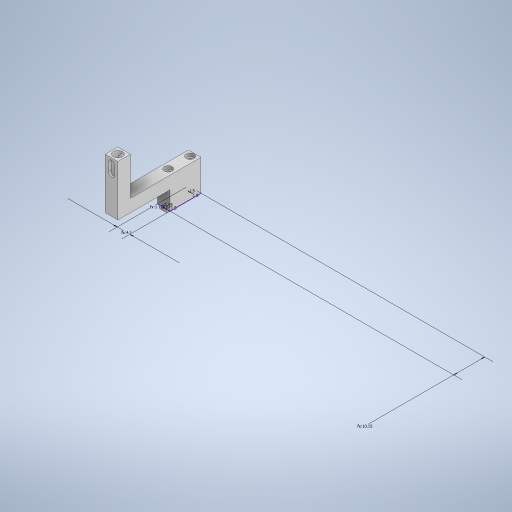
# Autodesk Inventor part: original_holder
Saved by Autodesk Inventor 2024 (Build 280153000, 153)
## iProperties
Created: 2023-05-03
Part Number: original_holder
Material: Generic
Document SubType Name: Modeling
Designer: Rober
Mass: 538.313 g
Surface Area: 676.575 cm^2
Volume: 538.313 cm^3
Density: 1 g/cm^3
Appearance: Default
Author: Rober
Autodesk Inventor part; units mm, degrees
ref_plane "YZ Plane" through (0, 0, 0) normal (1, 0, 0) x (0, 1, 0)
ref_plane "XZ Plane" through (0, 0, 0) normal (0, 1, 0) x (-1, 0, 0)
ref_plane "XY Plane" through (0, 0, 0) normal (0, 0, 1) x (1, 0, 0)
sketch "Sketch1" plane through (0, 0, 0) normal (0, 1, 0) x (-1, 0, 0)
  line L0 (-2.05, -5.575) -> (-6.15, -5.575)
  line L1 (-6.15, -5.575) -> (-6.15, 4.575)
  line L2 (-6.15, 4.575) -> (-2.05, 4.575)
  line L3 (-2.05, 4.575) -> (-2.05, -5.575)
  line L4 (-3.175, 4.575) -> (-5.025, 4.575)
  line L5 (-3.175, 4.575) -> (-3.175, -5.575)
  line L6 (-5.025, 4.575) -> (-5.025, -5.575)
  circle A0 centre (-4.1, 3.075) radius 0.75
  circle A1 centre (-4.1, -4.075) radius 0.75
  point P0 (-4.1, 4.575)
  point P1 (-4.1, -5.575)
  point P2 (-1.1679, -0.0702)
  point P3 (-4.1, 4.575)
  dimension "d13" = 4.1
  dimension "d14" = 10.15
  dimension "d44" = 1.85
  dimension "d45" = 1.125
  dimension "d46" = 1.5
  dimension "d47" = 1.5
  dimension "d48" = 1.5
  dimension "d49" = 1.5
  constraints: 14 end point, 4 point on line, 3 midpoint, 3 perpendicular, 2 centre point, 2 parallel, 1 horizontal
  measures "d13" distance of L0.start L0.end
  measures "d14" distance of point (-4.1, 4.575) point (-4.1, -5.575)
  measures "d44" distance of L4.start L4.end
  measures "d45" distance from line of L3 L4.start
  measures "d46" diameter of A0
  measures "d47" diameter of A1
  measures "d48" distance of point (-4.1, 4.575) A0.centre
  measures "d49" distance of point (-4.1, -5.575) A1.centre
extrude "Extrusion1" add sketch "Sketch1" along normal blind 10.15
sketch "Sketch11" plane through (2.05, 0, 4.575) normal (0, 0, 1) x (1, 0, 0)
  point P0 (-2.05, 0)
extrude "Extrusion6" add sketch "Sketch1" against normal blind 1 contours L0 L6 L2 L5
sketch "Sketch12" plane through (0, 10.15, 0) normal (0, 1, 0) x (1, 0, 0)
  circle A0 centre (4.0754, 4.0842) radius 1.265
  circle A1 centre (4.0754, -3.0807) radius 1.265
  point P0 (0, 0)
  dimension "d52" = 2.53
  dimension "d53" = 2.53
  constraints: 2 centre point
  measures "d52" diameter of A0
  measures "d53" diameter of A1
extrude "Extrusion7" cut sketch "Sketch12" against normal blind 1
sketch "Sketch13" plane through (2.05, 10.15, 4.575) normal (0, 0, 1) x (1, 0, 0)
  line L0 (0, 0) -> (0, -4.15)
  line L1 (0, -10.15) -> (0, 0) projected
  line L2 (0, -4.15) -> (4.1, -4.15)
  line L3 (4.1, -10.15) -> (4.1, 0) projected
  line L4 (4.1, 0) -> (4.1, -4.15)
  line L5 (0, 0) -> (4.1, 0)
  point P0 (-2.05, -10.15)
  dimension "d56" = 4.15
  constraints: 8 end point, 3 perpendicular, 2 point on line
  measures "d56" distance of L0.start L0.end
extrude "Extrusion8" add sketch "Sketch13" along normal blind 17
sketch "Sketch14" plane through (0, 10.15, 0) normal (0, 1, 0) x (1, 0, 0)
  line L0 (6.15, 5.575) -> (6.15, -21.575) projected
  line L1 (6.15, -21.575) -> (6.15, -17.465)
  line L2 (6.15, -17.465) -> (2.05, -17.465)
  line L3 (2.05, 5.575) -> (2.05, -21.575) projected
  line L4 (2.05, -21.575) -> (6.15, -21.575)
  point P0 (0, 0)
  dimension "d59" = 4.11
  constraints: 6 end point, 2 point on line, 1 parallel, 1 perpendicular
  measures "d59" distance of L0.end L1.end
extrude "Extrusion9" add sketch "Sketch14" along normal blind 12.4
sketch "Sketch15" plane through (2.05, 10.15, 21.575) normal (0, 0, 1) x (1, 0, 0)
  line L0 (2.05, 10.7632) -> (2.05, 7.9632) construction
  line L1 (4.1, 0) -> (4.1, 12.4) projected
  line L2 (1.05, 10.7632) -> (1.05, 7.9632)
  line L3 (3.05, 7.9632) -> (3.05, 10.7632)
  arc A0 (3.05, 10.7632) -> (1.05, 10.7632) centre (2.05, 10.7632) ccw
  arc A1 (1.05, 7.9632) -> (3.05, 7.9632) centre (2.05, 7.9632) ccw
  point P0 (-2.05, -10.15)
  point P1 (2.05, 9.3632)
  dimension "d62" = 1.4
  dimension "d63" = 2
  dimension "d64" = 2.05
  constraints: 8 end point, 4 point on circle, 4 tangent, 2 centre point, 2 parallel, 1 midpoint
  measures "d62" distance of point (2.05, 9.363) L0.end
  measures "d63" diameter of A1
  measures "d64" distance from line of L1 point (2.05, 9.363)
extrude "Extrusion10" cut sketch "Sketch15" against normal through all
sketch "Sketch16" plane through (0, 22.55, 0) normal (0, 1, 0) x (1, 0, 0)
  circle A0 centre (4.1, -19.52) radius 1.5
  line L0 (2.05, -21.575) -> (6.15, -21.575) projected
  line L1 (6.15, -21.575) -> (6.15, -17.465) projected
  point P0 (0, 0)
  point P1 (4.1, -21.575)
  dimension "d67" = 3
  dimension "d68" = 2.055
  dimension "d69" = 2.05
  constraints: 1 centre point, 1 midpoint
  measures "d67" diameter of A0
  measures "d68" distance of point (4.1, -21.575) A0.centre
  measures "d69" distance from line of L1 A0.centre
extrude "Extrusion11" cut sketch "Sketch16" against normal blind 10
equation "\"d13\" = base_width"
equation "\"d14\" = base_length"
equation "\"d45\" = -0.5 * d44 + 0.5 * d13"
equation "\"d4\" = base_length"
equation "\"base_width\" = 4.1"
equation "\"base_length\" = 10.15"
equation "\"base_screw_diameter\" = 1.5"
equation "\"base_screw_spacing_edge\" = 8.5"
body "Solid1"
